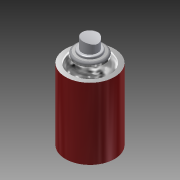
# Autodesk Inventor part: SprayCan77mm
Saved by Autodesk Inventor 2014 SP1 (Build 180222100, 222)
## iProperties
Created: 2017-02-11
Part Number: SprayCan77mm
Material: Generic
Document SubType Name: Modeling
Designer: danielsikar
Density: 1 g/cm^3
Appearance: Default
Author: danielsikar
Autodesk Inventor part; units mm, degrees
ref_plane "XZ Plane" through (0, 0, 0) normal (0, 1, 0) x (-1, 0, 0)
sketch "Sketch1" plane through (0, 0, 0) normal (0, 0, 1) x (1, 0, 0)
  circle A0 centre (0, 0) radius 26.5
  dimension "d0" = 53
  constraints: 1 centre point, 1 coincident
  measures "d0" diameter of A0
extrude "Extrusion1" add sketch "Sketch1" along normal blind 105
sketch "Sketch2" plane through (0, 0, 0) normal (0, 1, 0) x (-1, 0, 0)
  line L0 (6.5, 97) -> (21.5, 97)
  line L1 (21.5, 97) -> (21.5, 105)
  line L2 (14, 112.160816) -> (6.5, 112.160816)
  line L3 (6.5, 105) -> (6.5, 97)
  line L4 (26.5, 0) -> (26.5, 105) construction
  line L5 (0, -19.756358) -> (0, 218.345658) construction
  line L6 (21.5, 105) -> (0, 105)
  line L7 (0, 105) -> (0, 112.160816)
  line L8 (0, 112.160816) -> (14, 112.160816)
  line L9 (14, 122.762224) -> (14, 96.929674) construction
  arc A0 (21.5, 105) -> (14, 112.160816) centre (9.326615, 99.758035) ccw construction
  arc A1 (21.5, 105) -> (14, 112.160816) centre (9.326615, 99.758035) ccw
  line L10 (0, -67.376762) -> (0, 265.966062)
  point P0 (0, 0)
  dimension "d4" = 8
  dimension "d5" = 5
  constraints: 18 end point, 4 parallel, 4 point on circle, 3 point on line, 2 centre point, 2 horizontal, 2 perpendicular, 1 concentric
  measures "d4" distance of L1.end L0.end
  measures "d5" distance between parallel lines of L4 L1
revolve "Revolution1" add sketch "Sketch2" angle 360 about axis through (0, 0, -10) along (0, 0, 1) contours L6 L7 L8 L2 A1
sketch "Sketch3" plane through (0, 0, 112.160816) normal (0, 0, 1) x (1, 0, 0)
  circle A0 centre (0, 0) radius 14 projected
  circle A1 centre (0, 0) radius 16
  dimension "d8" = 32
  constraints: 1 centre point, 1 coincident
  measures "d8" diameter of A1
extrude "Extrusion2" add sketch "Sketch3" along normal blind 4 contours A0 | A1
sketch "Sketch4" plane through (0, 0, 116.160816) normal (0, 0, 1) x (1, 0, 0)
  circle A0 centre (0, 0) radius 16 projected
  circle A1 centre (0, 0) radius 11.25
  dimension "d11" = 22.5
  constraints: 1 centre point, 1 coincident
  measures "d11" diameter of A1
extrude "Extrusion3" add sketch "Sketch4" along normal blind 2.5 contours A1
sketch "Sketch5" plane through (0, 0, 118.660816) normal (0, 0, 1) x (1, 0, 0)
  circle A0 centre (0, 0) radius 11.25 projected
  circle A1 centre (0, 0) radius 8.5
  dimension "d14" = 17
  constraints: 1 centre point, 1 coincident
  measures "d14" diameter of A1
extrude "Extrusion4" add sketch "Sketch5" along normal blind 11 contours A1
ref_plane "Work Plane1" through (8.5, 0, 0) normal (1, 0, 0) x (0, 1, 0)
sketch "Sketch6" plane through (8.5, 0, 0) normal (1, 0, 0) x (0, 1, 0)
  line L0 (8.5, 129.660816) -> (-8.5, 129.660816) construction
  line L1 (11.25, 118.660816) -> (-11.25, 118.660816) construction
  line L2 (-11.850613, 127.160816) -> (16.091514, 127.160816) construction
  line L3 (-8.5, 118.660816) -> (-8.5, 129.660816) construction
  line L4 (8.5, 118.660816) -> (8.5, 129.660816) construction
  arc A0 (-8.5, 129.660816) -> (8.5, 129.660816) centre (0, 142.860816) ccw
  line L5 (-8.5, 129.660816) -> (8.5, 129.660816)
  point P0 (0, 0)
  dimension "d18" = 8.5
  constraints: 4 end point, 2 point on circle, 1 centre point, 1 collinear, 1 parallel, 1 tangent
  measures "d18" distance between parallel lines of L2 L1
ref_plane "Work Plane2" through (-8.5, 0, 0) normal (1, 0, 0) x (0, 1, 0)
sketch "Sketch7" plane through (-8.5, 0, 0) normal (1, 0, 0) x (0, 1, 0)
  line L0 (8.5, 118.660816) -> (8.5, 129.660816) construction
  line L1 (-8.5, 118.660816) -> (-8.5, 129.660816) construction
  line L2 (11.25, 118.660816) -> (-11.25, 118.660816) construction
  line L3 (10.28234, 132.160816) -> (-15.326143, 132.160816) construction
  line L4 (8.5, 128.85356) -> (8.5, 132.770152) construction
  line L5 (-8.5, 128.418383) -> (-8.5, 133.238804) construction
  line L6 (8.5, 132.160816) -> (-8.5, 132.160816)
  line L7 (14.5, 124.804712) -> (14.5, 141.766568) construction
  line L8 (-14.5, 142.728943) -> (-14.5, 126.729462) construction
  line L9 (18.190676, 132.160816) -> (-22.229061, 132.160816) construction
  arc A0 (-14.5, 132.160816) -> (14.5, 132.160816) centre (0, 172.960816) ccw
  line L10 (14.5, 132.160816) -> (-14.5, 132.160816)
  point P0 (0, 0)
  dimension "d22" = 6
  dimension "d23" = 6
  constraints: 16 end point, 11 point on line, 3 parallel, 2 collinear, 2 perpendicular, 2 point on circle, 1 centre point
  measures "d22" distance between parallel lines of L7 L0
  measures "d23" distance between parallel lines of L8 L1
sketch "Sketch6 outline for Loft1" plane through (8.5, 0, 0) normal (1, 0, 0) x (0, 1, 0)
  line L0 (8.5, 129.660816) -> (-8.5, 129.660816)
  arc A0 (-8.5, 129.660816) -> (8.5, 129.660816) centre (0, 142.860816) ccw
sketch "Sketch7 outline for Loft1" plane through (-8.5, 0, 0) normal (1, 0, 0) x (0, 1, 0)
  line L0 (14.5, 132.160816) -> (-14.5, 132.160816)
  arc A0 (-14.5, 132.160816) -> (14.5, 132.160816) centre (0, 172.960816) ccw
loft "Loft1" cut profiles "Sketch6 outline for Loft1", "Sketch7 outline for Loft1"
fillet "Fillet1" radius 2 1 edges at (-16, 0, 116.1608)
fillet "Fillet2" radius 1 1 edges at (-11.25, 0, 118.6608)
sketch "Sketch8" plane through (0, 0, 0) normal (0, 0, -1) x (-1, 0, 0)
  circle A0 centre (0, 0) radius 26.5 projected
extrude "Extrusion5" cut sketch "Sketch8" against normal blind 28
body "Solid1"
